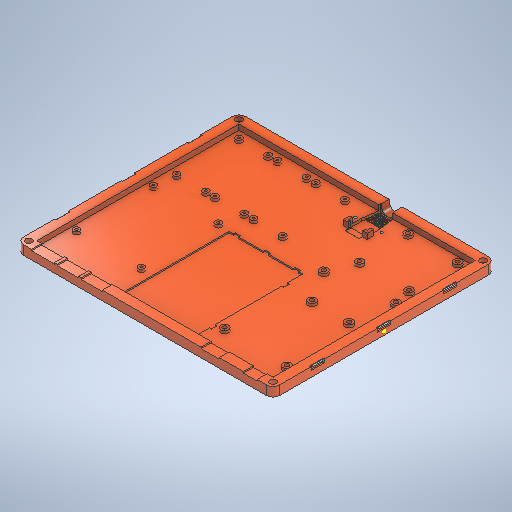
# Autodesk Inventor part: Electronic Base - Layered
Saved by Autodesk Inventor 2025.2 (Build 292293000, 293)
## iProperties
Created: 2025-02-05
Part Number: Electronic Base - Layered
Material: Generic
Document SubType Name: Modeling
Designer: caomi
Density: 1 g/cm^3
Appearance: Default
Author: caomi
Autodesk Inventor part; units mm, degrees
ref_plane "YZ Plane" through (0, 0, 0) normal (1, 0, 0) x (0, 1, 0)
ref_plane "XZ Plane" through (0, 0, 0) normal (0, 1, 0) x (-1, 0, 0)
ref_plane "XY Plane" through (0, 0, 0) normal (0, 0, 1) x (1, 0, 0)
sketch "Sketch1" plane through (0, 0, 0) normal (0, 1, 0) x (-1, 0, 0)
  line L0 (193.34, 167.6) -> (0, 167.6)
  line L1 (0, 167.6) -> (0, 0)
  line L2 (0, 0) -> (193.34, 0)
  line L3 (193.34, 0) -> (193.34, 167.6)
  line L4 (183.84, 74.1) -> (127.84, 74.1) construction
  line L5 (127.84, 74.1) -> (127.84, 159.1) construction
  line L6 (127.84, 159.1) -> (183.84, 159.1) construction
  line L7 (183.84, 159.1) -> (183.84, 74.1) construction
  circle A0 centre (180.34, 77.6) radius 0.9
  circle A1 centre (180.34, 135.6) radius 0.9
  circle A2 centre (131.34, 77.6) radius 0.9
  circle A3 centre (131.34, 135.6) radius 0.9
  line L8 (0, 0) -> (-136.9444, 0) construction
  line L9 (0, 0) -> (0, -49.9102) construction
  circle A4 centre (180.34, 77.6) radius 2.4
  circle A5 centre (180.34, 135.6) radius 2.4
  circle A6 centre (131.34, 77.6) radius 2.4
  circle A7 centre (131.34, 135.6) radius 2.4
  line L10 (185.84, 7.5) -> (7.5, 7.5)
  line L11 (7.5, 7.5) -> (7.5, 160.1)
  line L12 (7.5, 160.1) -> (185.84, 160.1)
  line L13 (185.84, 160.1) -> (185.84, 7.5)
  line L14 (62.84, 57.5) -> (9.5, 57.5) construction
  line L15 (9.5, 57.5) -> (9.5, 159.1) construction
  line L16 (9.5, 159.1) -> (62.84, 159.1) construction
  line L17 (62.84, 159.1) -> (62.84, 57.5) construction
  circle A8 centre (60.3, 68.93) radius 3.05
  circle A9 centre (60.3, 68.93) radius 1.55
  circle A10 centre (45.06, 93.06) radius 3.05
  circle A11 centre (45.06, 93.06) radius 1.55
  circle A12 centre (60.3, 143.86) radius 1.55
  circle A13 centre (17.12, 93.06) radius 3.05
  circle A14 centre (60.3, 143.86) radius 3.05
  circle A15 centre (17.12, 93.06) radius 1.55
  circle A16 centre (12.04, 62.58) radius 3.05
  circle A17 centre (12.04, 62.58) radius 1.55
  circle A18 centre (12.04, 145.13) radius 3.05
  circle A19 centre (12.04, 145.13) radius 1.55
  line L18 (122.9704, 77.92) -> (68.2204, 77.92) construction
  line L19 (68.2204, 77.92) -> (68.2204, 159.6) construction
  line L20 (68.2204, 159.6) -> (122.9704, 159.6) construction
  line L21 (122.9704, 159.6) -> (122.9704, 77.92) construction
  line L22 (55.5, 9.5) -> (12.5, 9.5) construction
  line L23 (12.5, 9.5) -> (12.5, 52.5) construction
  line L24 (12.5, 52.5) -> (55.5, 52.5) construction
  line L25 (55.5, 52.5) -> (55.5, 9.5) construction
  line L26 (180.84, 63.5) -> (154.84, 63.5) construction
  line L27 (154.84, 63.5) -> (154.84, 12.5) construction
  line L28 (154.84, 12.5) -> (180.84, 12.5) construction
  line L29 (180.84, 12.5) -> (180.84, 63.5) construction
  circle A20 centre (178.84, 14.5) radius 0.9
  circle A21 centre (178.84, 14.5) radius 2.4
  circle A22 centre (156.84, 14.5) radius 2.4
  circle A23 centre (156.84, 14.5) radius 0.9
  circle A24 centre (178.84, 61.5) radius 2.4
  circle A25 centre (178.84, 61.5) radius 0.9
  circle A26 centre (156.84, 61.5) radius 0.9
  circle A27 centre (156.84, 61.5) radius 2.4
  line L30 (125.84, 12.5) -> (151.84, 12.5) construction
  circle A28 centre (127.84, 14.5) radius 0.9
  circle A29 centre (149.84, 14.5) radius 0.9
  circle A30 centre (127.84, 14.5) radius 2.4
  circle A31 centre (149.84, 14.5) radius 2.4
  circle A32 centre (127.84, 61.5) radius 0.9
  circle A33 centre (127.84, 61.5) radius 2.4
  line L31 (125.84, 63.5) -> (125.84, 12.5) construction
  line L32 (151.84, 63.5) -> (125.84, 63.5) construction
  circle A34 centre (149.84, 61.5) radius 2.4
  line L33 (151.84, 12.5) -> (151.84, 63.5) construction
  circle A35 centre (149.84, 61.5) radius 0.9
  line L34 (96.84, 12.5) -> (122.84, 12.5) construction
  circle A36 centre (98.84, 14.5) radius 0.9
  circle A37 centre (120.84, 14.5) radius 0.9
  circle A38 centre (98.84, 14.5) radius 2.4
  circle A39 centre (120.84, 14.5) radius 2.4
  circle A40 centre (98.84, 61.5) radius 0.9
  circle A41 centre (98.84, 61.5) radius 2.4
  line L35 (96.84, 63.5) -> (96.84, 12.5) construction
  line L36 (122.84, 63.5) -> (96.84, 63.5) construction
  circle A42 centre (120.84, 61.5) radius 2.4
  line L37 (122.84, 12.5) -> (122.84, 63.5) construction
  circle A43 centre (120.84, 61.5) radius 0.9
  line L38 (67.7204, 77.42) -> (123.4704, 77.42)
  line L39 (123.4704, 77.42) -> (123.4704, 160.1)
  line L40 (123.4704, 160.1) -> (67.7204, 160.1)
  line L41 (67.7204, 160.1) -> (67.7204, 77.42)
  line L42 (97.5954, 77.42) -> (93.5954, 77.42)
  line L43 (93.5954, 77.42) -> (93.5954, 75.92)
  line L44 (93.5954, 75.92) -> (97.5954, 75.92)
  line L45 (97.5954, 75.92) -> (97.5954, 77.42)
  line L46 (116.2954, 75.92) -> (120.2954, 75.92)
  line L47 (120.2954, 75.92) -> (120.2954, 77.42)
  line L48 (116.2954, 77.42) -> (116.2954, 75.92)
  line L49 (70.8954, 75.92) -> (74.8954, 75.92)
  line L50 (74.8954, 75.92) -> (74.8954, 77.42)
  line L51 (70.8954, 77.42) -> (70.8954, 75.92)
  line L52 (67.7204, 143.7) -> (66.2204, 143.7)
  line L53 (66.2204, 143.7) -> (66.2204, 147.7)
  line L54 (66.2204, 147.7) -> (67.7204, 147.7)
  line L55 (67.7204, 147.7) -> (67.7204, 143.7)
  line L56 (67.7204, 89.17) -> (66.2204, 89.17)
  line L57 (66.2204, 89.17) -> (66.2204, 93.17)
  line L58 (66.2204, 93.17) -> (67.7204, 93.17)
  circle A44 centre (15.371, 12.82) radius 1.4
  circle A45 centre (15.371, 12.82) radius 2.9
  circle A46 centre (52.744, 12.82) radius 2.9
  circle A47 centre (52.744, 12.82) radius 1.4
  circle A48 centre (15.371, 49.557) radius 1.4
  circle A49 centre (15.371, 49.557) radius 2.9
  circle A50 centre (52.744, 49.557) radius 2.9
  circle A51 centre (52.744, 49.557) radius 1.4
  point P0 (183.84, 116.6)
  point P1 (9.5, 108.3)
  point P2 (1.5544, 63)
  point P3 (2.0056, 63)
  point P4 (82.8344, 63)
  point P5 (83.2856, 63)
  point P6 (36.17, 159.1)
  point P7 (95.5954, 75.92)
  point P8 (95.5954, 77.42)
  point P9 (118.2954, 75.92)
  point P10 (72.8954, 75.92)
  point P11 (66.2204, 145.7)
  point P12 (34, 9.5)
  point P13 (66.2204, 91.17)
  point P14 (70.8954, 77.42)
  point P15 (74.8954, 77.42)
  point P16 (93.5954, 77.42)
  point P17 (116.2954, 77.42)
  point P18 (120.2954, 77.42)
  dimension "d10" = 1.8
  dimension "d49" = 53.34
  dimension "d59" = 7.5
  dimension "d62" = 3.1
  dimension "d63" = 1.5
  dimension "d73" = 7.5
  dimension "d79" = 7.5
  dimension "d82" = 2.54
  dimension "d83" = 15.24
  dimension "d84" = 90.17
  dimension "d85" = 96.52
  dimension "d86" = 50.8
  dimension "d87" = 66.04
  dimension "d88" = 17.78
  dimension "d89" = 45.72
  dimension "d90" = 13.97
  dimension "d91" = 85
  dimension "d92" = 58
  dimension "d95" = 1.5
  dimension "d96" = 3.5
  dimension "d97" = 3.5
  dimension "d98" = 3.5
  dimension "d99" = 56
  dimension "d102" = 7.5
  dimension "d103" = 65
  dimension "d121" = 54.75
  dimension "d122" = 81.68
  dimension "d123" = 1
  dimension "d124" = 43
  dimension "d131" = 51
  dimension "d134" = 101.6
  dimension "d135" = 26
  dimension "d136" = 1.8
  dimension "d138" = 2
  dimension "d139" = 2
  dimension "d140" = 24
  dimension "d141" = 49
  dimension "d144" = 29
  dimension "d149" = 0.5
  dimension "d150" = 4
  dimension "d151" = 1.5
  dimension "d154" = 22.7
  dimension "d160" = 11.9
  dimension "d161" = 5
  dimension "d165" = 54.53
  dimension "d172" = 5
  dimension "d173" = 5
  dimension "d174" = 2
  dimension "d176" = 2.8
  dimension "d178" = 2
  dimension "d179" = 3.32
  dimension "d180" = 2.871
  dimension "d181" = 40.244
  dimension "d182" = 40.057
  dimension "d183" = 5
  dimension "d184" = 2
  dimension "d277" = 1.5
  dimension "d278" = 1.5
  constraints: 118 end point, 52 centre point, 28 equal radius, 22 coincident, 20 parallel, 13 perpendicular, 12 horizontal, 9 vertical alignment, 7 horizontal alignment, 7 midpoint, 3 collinear, 2 point on line, 2 vertical, 74 other
  measures "d10" diameter of A0
  measures "d49" distance of L15.end L16.end
  measures "d59" distance between parallel lines of L13 L3
  measures "d62" diameter of A9
  measures "d63" radial gap between concentric circles of A8 A9
  measures "d73" distance between parallel lines of L0 L12
  measures "d79" distance between parallel lines of L2 L10
  measures "d82" distance from line of L17 A12.centre
  measures "d83" distance from line of L16 A12.centre
  measures "d84" distance from line of L16 A9.centre
  measures "d85" distance from line of L16 A16.centre
  measures "d86" distance from line of L17 A17.centre
  measures "d87" distance from line of L16 A10.centre
  measures "d88" distance from line of L17 A10.centre
  measures "d89" distance from line of L17 A15.centre
  measures "d90" distance from line of L16 A18.centre
  measures "d91" distance of L4.end L5.end
  measures "d92" distance of A3.centre A2.centre
  measures "d95" radial gap between concentric circles of A4 A0
  measures "d96" distance from line of L4 A2.centre
  measures "d97" distance from line of L7 A0.centre
  measures "d98" distance from line of L5 A2.centre
  measures "d99" distance between parallel lines of L7 L5
  measures "d102" distance between parallel lines of L1 L11
  measures "d103" distance between parallel lines of L17 L5
  measures "d121" distance of L19.end L20.end
  measures "d122" distance of L18.end L19.end
  measures "d123" distance between parallel lines of L12 L16
  measures "d124" distance of L22.end L23.end
  measures "d131" distance of L28.end L26.start
  measures "d134" distance of L14.end L15.end
  measures "d135" distance of L27.end L28.end
  measures "d136" diameter of A20
  measures "d138" distance from line of L29 A20.centre
  measures "d139" distance from line of A20.centre L28
  measures "d140" distance from line of L29 A22.centre
  measures "d141" distance from line of L28 A24.centre
  measures "d144" distance of A22.centre A30.centre
  measures "d149" distance between parallel lines of L19 L41
  measures "d150" distance of L43.end L44.end
  measures "d151" distance between parallel lines of L38 L44
  measures "d154" distance of point (95.595, 75.92) point (118.295, 75.92)
  measures "d160" distance between parallel lines of L20 L54
  measures "d161" distance between parallel lines of L24 L14
  measures "d165" distance of L52.start L56.start
  measures "d172" distance between parallel lines of L13 L29
  measures "d173" distance between parallel lines of L10 L28
  measures "d174" distance between parallel lines of L7 L13
  measures "d176" diameter of A44
  measures "d178" vertical distance of L10.end L22.end
  measures "d179" distance from line of L22 A44.centre
  measures "d180" distance from line of L23 A44.centre
  measures "d181" distance from line of L23 A46.centre
  measures "d182" distance from line of L22 A48.centre
  measures "d183" distance between parallel lines of L11 L23
  measures "d184" horizontal distance of L11.end L15.end
  measures "d277" radial gap between concentric circles of A20 A21
  measures "d278" radial gap between concentric circles of A44 A45
extrude "Extrusion1" add sketch "Sketch1" against normal blind 3 contours L3 L2 L1 L0 | A0 | A1 | A2 | A3 | A4 | A5 | A6 | A7 | L10 L11 L12 L41 L54 L53 L52 L58 L57 L56 L38 L51 L49 L50 L43 L44 L45 L48 L46 L47 L39 L13 | L39 L38 L41 L12 | L41 L52 L53 L54 | L47 L46 L48 L38 | L41 L56 L57 L58 | L45 L44 L43 L38 | L50 L49 L51 L38 | A8 | A9 | A10 | A11 | A12 | A13 | A14 | A15 | A16 | A17 | A18 | A19 | A20 | A21 | A22 | A23 | A24 | A25 | A26 | A27 | A28 | A29 | A30 | A31 | A32 | A33 | A34 | A35 | A36 | A37 | A38 | A39 | A40 | A41 | A42 | A43 | A44 | A45 | A46 | A47 | A48 | A49 | A50 | A51
extrude "Extrusion2" add sketch "Sketch1" along normal blind 4 contours L3 L2 L1 L0
extrude "Extrusion5" cut sketch "Sketch1" against normal blind 1 contours L39 L38 L41 L12 | L41 L52 L53 L54 | L47 L46 L48 L38 | L41 L56 L57 L58 | L45 L44 L43 L38 | L50 L49 L51 L38
extrude "Extrusion3" add sketch "Sketch1" along normal blind 2 contours A4 | A5 | A6 | A7 | A8 | A10 | A13 | A14 | A16 | A18 | A21 | A22 | A24 | A27 | A30 | A31 | A33 | A34 | A38 | A39 | A41 | A42 | A45 | A46 | A49 | A50
fillet "Fillet1" radius 5 4 edges at (-193.34, 0.5, 0) (0, 0.5, 167.6) (-193.34, 0.5, 167.6) (0, 0.5, 0)
sketch "Sketch2" plane through (0, 4, 0) normal (0, 1, 0) x (1, 0, 0)
  line L0 (-188.34, -167.6) -> (-5, -167.6) projected
  line L1 (-7.5, -160.1) -> (-185.84, -160.1) projected
  line L2 (-182.34, -160.1) -> (-164.94, -160.1)
  line L3 (-164.94, -160.1) -> (-164.94, -167.6)
  line L4 (-164.94, -167.6) -> (-182.34, -167.6)
  line L5 (-182.34, -167.6) -> (-182.34, -160.1)
  line L6 (-162.84, -160.1) -> (-146.74, -160.1)
  line L7 (-146.74, -160.1) -> (-146.74, -167.6)
  line L8 (-146.74, -167.6) -> (-162.84, -167.6)
  line L9 (-162.84, -167.6) -> (-162.84, -160.1)
  line L10 (-144.84, -160.1) -> (-128.84, -160.1)
  line L11 (-128.84, -160.1) -> (-128.84, -167.6)
  line L12 (-128.84, -167.6) -> (-144.84, -167.6)
  line L13 (-144.84, -167.6) -> (-144.84, -160.1)
  line L14 (-54.34, -160.1) -> (-40.7, -160.1)
  line L15 (-40.7, -160.1) -> (-40.7, -167.6)
  line L16 (-40.7, -167.6) -> (-54.34, -167.6)
  line L17 (-54.34, -167.6) -> (-54.34, -160.1)
  line L18 (-183.84, -159.1) -> (-183.84, -74.1) construction
  line L19 (-62.84, -159.1) -> (-62.84, -57.5) construction
  line L20 (-22.34, -160.1) -> (-12.01, -160.1)
  line L21 (-12.01, -160.1) -> (-12.01, -167.6)
  line L22 (-12.01, -167.6) -> (-22.34, -167.6)
  line L23 (-22.34, -167.6) -> (-22.34, -160.1)
  point P0 (0, 0)
  point P1 (-128.84, -160.1)
  point P2 (-146.74, -160.1)
  point P3 (-164.94, -160.1)
  point P4 (-12.01, -163.85)
  point P5 (-12.01, -160.1)
  dimension "d104" = 17.4
  dimension "d107" = 16.1
  dimension "d109" = 16
  dimension "d113" = 13.64
  dimension "d114" = 1.5
  dimension "d115" = 21
  dimension "d116" = 39
  dimension "d117" = 8.5
  dimension "d118" = 40.5
  dimension "d119" = 10.33
  constraints: 40 end point, 10 parallel, 10 point on line, 5 horizontal, 5 perpendicular, 1 midpoint
  measures "d104" distance of L3.end L4.end
  measures "d107" distance of L7.end L8.end
  measures "d109" distance between parallel lines of L11 L13
  measures "d113" distance between parallel lines of L15 L17
  measures "d114" distance between parallel lines of L18 L5
  measures "d115" distance between parallel lines of L18 L9
  measures "d116" distance between parallel lines of L18 L13
  measures "d117" distance between parallel lines of L19 L17
  measures "d118" distance between parallel lines of L19 L23
  measures "d119" distance from line of point (-12.01, -163.85) L23
extrude "Extrusion4" cut sketch "Sketch2" against normal blind 1 contours L5 L1 L3 L0 | L9 L1 L7 L0 | L13 L1 L11 L0 | L17 L1 L15 L0 | L23 L1 L21 L0
ref_plane "Work Plane5" through (-188.34, 0, 167.6) normal (0, 0, 1) x (1, 0, 0)
sketch "Sketch3" plane through (-188.34, 0, 167.6) normal (0, 0, 1) x (1, 0, 0)
  line L0 (-3, 2.5) -> (-4, 1.5)
  line L1 (-3, 2.5) -> (-4, 3.5)
  line L2 (-3, 2.5) -> (-4, 2.5) construction
  line L3 (-5, -3) -> (-5, 4) projected
  line L4 (-5, 4) -> (-4, 4)
  line L5 (-4, 4) -> (-4, 1.5)
  line L6 (-4, 1.5) -> (-5, 1.5)
  line L7 (-5, 1.5) -> (-5, 4)
  point P0 (188.34, 0)
  point P1 (-4, 3.1514)
  dimension "d201" = 1
  dimension "d210" = 2.5
  dimension "d211" = 1
  dimension "d222" = 45
  constraints: 14 end point, 2 horizontal, 2 parallel, 2 point on line, 1 perpendicular, 1 other
  measures "d201" distance of L0.start L2.end
  measures "d210" distance between parallel lines of L4 L6
  measures "d211" distance of L3.end L4.end
  measures "d222" angle of L0 L5
ref_plane "Work Plane2" through (-188.34, 0, 83.8) normal (0, 0, 1) x (1, 0, 0)
extrude "Extrusion6" cut sketch "Sketch3" along normal mid plane 10 from surface at -83.8
pattern_linear "Rectangular Pattern2" count 3 spacing 50 along (0, 0, -1) of "Extrusion6" first direction both ways yes
ref_plane "Work Plane3" through (-96.67, 0, 5) normal (-1, 0, 0) x (0, 0, 1)
mirror "Mirror2" about plane through (-96.67, 0, 5) normal (-1, 0, 0) of "Extrusion6", "Rectangular Pattern2"
sketch "Sketch4" plane through (0, 4, 0) normal (0, 1, 0) x (1, 0, 0)
  line L0 (-190.4854, -1.65) -> (-187.1946, -1.65)
  line L1 (-187.1946, -1.65) -> (-185.5491, -4.5)
  line L2 (-185.5491, -4.5) -> (-187.1946, -7.35)
  line L3 (-187.1946, -7.35) -> (-190.4854, -7.35)
  line L4 (-190.4854, -7.35) -> (-192.1309, -4.5)
  line L5 (-192.1309, -4.5) -> (-190.4854, -1.65)
  line L6 (-193.34, -5) -> (-193.34, -162.6) projected
  line L7 (-5, 0) -> (-188.34, 0) projected
  point P0 (0, 0)
  point P1 (-188.84, -4.5)
  point P2 (-193.34, -28.8)
  dimension "d205" = 5.7
  dimension "d206" = 4.5
  dimension "d207" = 4.5
  constraints: 12 end point, 1 horizontal, 13 other
  measures "d205" distance between parallel lines of L0 L3
  measures "d206" distance from line of L6 point (-188.84, -4.5)
  measures "d207" distance from line of L7 point (-188.84, -4.5)
extrude "Extrusion7" cut sketch "Sketch4" along normal blind 1 from surface at -7
hole "Hole1" at (-188.84, 4, 4.5) direction (0, -1, 0) diameter 3 end through all counterbore diameter 5 counterbore depth 3.2
sketch "Sketch5" plane through (-188.34, 0, 83.8) normal (0, 0, 1) x (1, 0, 0)
  point P0 (188.34, 0)
mirror "Mirror3" about plane through (-96.67, 0, 5) normal (-1, 0, 0) of "Hole1", "Extrusion7"
mirror "Mirror4" about plane through (-188.34, 0, 83.8) normal (0, 0, 1) of "Hole1", "Extrusion7", "Mirror3"
sketch "Sketch6" plane through (0, 4, 0) normal (0, 1, 0) x (1, 0, 0)
  line L0 (-80.25, -6) -> (-69.75, -6)
  line L1 (-69.75, -6) -> (-68, -19)
  line L2 (-82, -19) -> (-80.25, -6)
  line L3 (-75, 7.1666) -> (-75, -22.0458) construction
  line L4 (-69.5346, -7.6) -> (-80.4654, -7.6)
  line L5 (-69.4269, -8.4) -> (-80.5731, -8.4)
  line L6 (-69.2654, -9.6) -> (-80.7346, -9.6)
  line L7 (-69.1577, -10.4) -> (-80.8423, -10.4)
  line L8 (-68.9962, -11.6) -> (-81.0038, -11.6)
  line L9 (-68.8885, -12.4) -> (-81.1115, -12.4)
  line L10 (-68.7269, -13.6) -> (-81.2731, -13.6)
  line L11 (-68.35, -16.4) -> (-81.65, -16.4)
  line L12 (-68.4577, -15.6) -> (-81.5423, -15.6)
  line L13 (-68, -19) -> (-68, -28.5)
  line L14 (-82, -28.5) -> (-82, -19)
  line L15 (0, -28.8) -> (0, -5) projected
  line L16 (-5, 0) -> (-188.34, 0) projected
  line L17 (-68.6192, -14.4) -> (-81.3808, -14.4)
  line L18 (-69.75, -28.5) -> (-69.75, -33)
  line L19 (-69.75, -33) -> (-80.25, -33)
  line L20 (-80.25, -33) -> (-80.25, -28.5)
  line L21 (-68.1885, -17.6) -> (-81.8115, -17.6)
  line L22 (-68.0808, -18.4) -> (-81.9192, -18.4)
  line L23 (-68, -28.5) -> (-69.75, -28.5)
  line L24 (-80.25, -28.5) -> (-82, -28.5)
  line L25 (-80.25, -28.5) -> (-69.75, -28.5)
  line L26 (-82, -25.5) -> (-84, -25.5)
  line L27 (-84, -25.5) -> (-84, -30.5)
  line L28 (-84, -30.5) -> (-80.5, -30.5)
  line L29 (-80.5, -30.5) -> (-80.5, -28.5)
  line L30 (-68, -25.5) -> (-66, -25.5)
  line L31 (-66, -25.5) -> (-66, -30.5)
  line L32 (-66, -30.5) -> (-69.5, -30.5)
  line L33 (-69.5, -30.5) -> (-69.5, -28.5)
  point P0 (0, 0)
  dimension "d223" = 10.5
  dimension "d224" = 14
  dimension "d226" = 1.6
  dimension "d227" = 0.8
  dimension "d228" = 1.2
  dimension "d229" = 0.8
  dimension "d230" = 1.2
  dimension "d231" = 0.8
  dimension "d232" = 1.2
  dimension "d235" = 0.8
  dimension "d239" = 75
  dimension "d240" = 6
  dimension "d241" = 0.8
  dimension "d242" = 1.2
  dimension "d253" = 10.5
  dimension "d255" = 1.2
  dimension "d260" = 0.8
  dimension "d261" = 13
  dimension "d262" = 9.5
  dimension "d263" = 4.5
  dimension "d265" = 2
  dimension "d266" = 2
  dimension "d267" = 3
  dimension "d268" = 1.5
  constraints: 60 end point, 18 horizontal, 5 symmetric about line, 2 parallel, 2 perpendicular, 2 point on line, 2 vertical, 1 collinear, 32 other
  measures "d223" distance of L0.start L0.end
  measures "d224" distance of L14.end L13.start
  measures "d226" distance between parallel lines of L4 L0
  measures "d227" distance between parallel lines of L5 L4
  measures "d228" distance between parallel lines of L5 L6
  measures "d229" distance between parallel lines of L6 L7
  measures "d230" distance between parallel lines of L8 L7
  measures "d231" distance between parallel lines of L8 L9
  measures "d232" distance between parallel lines of L10 L9
  measures "d235" distance between parallel lines of L12 L11
  measures "d239" distance between parallel lines of L15 L3
  measures "d240" distance between parallel lines of L16 L0
  measures "d241" distance between parallel lines of L10 L17
  measures "d242" distance between parallel lines of L17 L12
  measures "d253" distance of L18.end L19.end
  measures "d255" distance between parallel lines of L21 L11
  measures "d260" distance between parallel lines of L21 L22
  measures "d261" vertical distance of L13.start L0.end
  measures "d262" distance of L13.start L13.end
  measures "d263" distance between parallel lines of L23 L19
  measures "d265" distance of L28.end L29.end
  measures "d266" distance of L26.start L26.end
  measures "d267" distance between parallel lines of L24 L26
  measures "d268" distance between parallel lines of L29 L14
extrude "Extrusion8" cut sketch "Sketch6" against normal blind 6 contours L0 L1 L4 L2 | L4 L1 L5 L2 | L5 L1 L6 L2 | L6 L1 L7 L2 | L7 L1 L8 L2 | L8 L1 L9 L2 | L9 L1 L10 L2 | L10 L1 L17 L2 | L17 L1 L12 L2 | L12 L1 L11 L2 | L11 L1 L21 L2 | L21 L1 L22 L2 | L22 L1 L13 L23 L25 L24 L14 L2 | L25 L18 L19 L20
extrude "Extrusion9" add sketch "Sketch6" along normal blind 0.5 from surface at -6 contours L4 L1 L5 L2 | L6 L1 L7 L2 | L8 L1 L9 L2 | L10 L1 L17 L2 | L12 L1 L11 L2
extrude "Extrusion10" add sketch "Sketch6" along normal blind 1 from surface at -5.5 contours L25 L18 L19 L20
sketch "Sketch7" plane through (-80.25, 4, 6) normal (0, 0, 1) x (1, 0, 0)
  circle A0 centre (5.25, -1) radius 5
  line L0 (0, -6) -> (10.5, -6) projected
  point P0 (80.25, -4)
  point P1 (5.25, -6)
  point P2 (5.25, -6)
  dimension "d249" = 5
  dimension "d250" = 10
  constraints: 2 midpoint, 1 centre point, 1 vertical alignment
  measures "d249" distance of point (5.25, -6) A0.centre
  measures "d250" diameter of A0
extrude "Extrusion11" cut sketch "Sketch7" against normal up to surface (6 mm away)
extrude "Extrusion13" add sketch "Sketch6" against normal up to surface (4 mm away) contours L14 L24 L29 L28 L27 L26 | L30 L31 L32 L33 L23 L13
sketch "Sketch8" plane through (0, 4, 0) normal (0, 1, 0) x (1, 0, 0)
  line L0 (-188.34, 0) -> (-5, 0) projected
  line L1 (-87.5, 0) -> (-62.5, 0)
  line L2 (-62.5, 0) -> (-62.5, -35)
  line L3 (-62.5, -35) -> (-87.5, -35)
  line L4 (-87.5, -35) -> (-87.5, 0)
  line L5 (-75, 7.1666) -> (-75, -22.0458) construction
  point P0 (0, 0)
  dimension "d256" = 25
  dimension "d257" = 35
  constraints: 8 end point, 2 parallel, 1 horizontal, 1 perpendicular, 1 point on line, 1 other
  measures "d256" distance between parallel lines of L4 L2
  measures "d257" distance of L1.end L2.end
extrude "DC Jack Test Fit" [suppressed]
fillet "Fillet2" radius 0.75 6 edges at (-2, 2.5, 33.8) (-2, 2.5, 83.8) (-2, 2.5, 133.8) (-191.34, 2.5, 33.8) (-191.34, 2.5, 83.8) (-191.34, 2.5, 133.8)
sketch "Sketch9" plane through (0, 0, 0) normal (0, 1, 0) x (1, 0, 0)
  circle A0 centre (-85, -20.5) radius 1
  circle A1 centre (-65, -20.5) radius 1
  line L0 (-75, 7.1666) -> (-75, -22.0458) construction
  line L1 (-69.75, -28.5) -> (-80.25, -28.5) projected
  point P0 (0, 0)
  dimension "d272" = 20
  dimension "d273" = 2
  dimension "d274" = 8
  constraints: 2 centre point, 1 equal radius, 1 horizontal alignment, 1 other
  measures "d272" distance of A0.centre A1.centre
  measures "d273" diameter of A0
  measures "d274" distance from line of L1 A0.centre
extrude "Extrusion14" cut sketch "Sketch9" against normal blind 10
ref_plane "Work Plane4" through (-96.67, 0, 5) normal (-1, 0, 0) x (0, 0, 1)
equation "\"board_border\" = 2"
equation "\"base_wall\" = 7.5"
body "Solid1"
